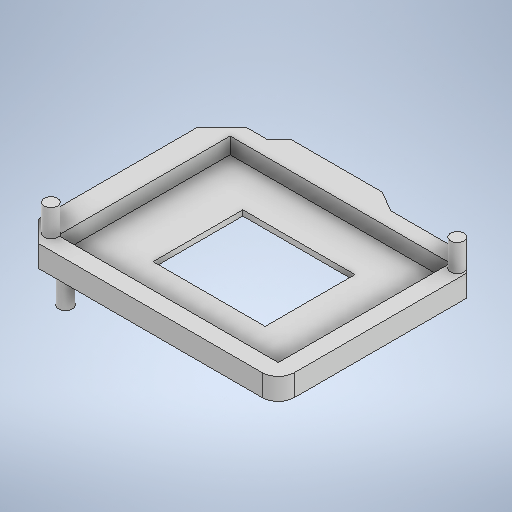
# Autodesk Inventor part: podstawka
Saved by Autodesk Inventor 2025.1 (Build 291241000, 241)
## iProperties
Created: 2024-10-24
Part Number: podstawka
Material: Ogólny
Document SubType Name: Modeling
Designer: PC
Density: 1 g/cm^3
Appearance: Domyślna
Author: PC
Autodesk Inventor part; units mm, degrees
ref_plane "YZ Plane" through (0, 0, 0) normal (1, 0, 0) x (0, 1, 0)
ref_plane "XZ Plane" through (0, 0, 0) normal (0, 1, 0) x (-1, 0, 0)
ref_plane "XY Plane" through (0, 0, 0) normal (0, 0, 1) x (1, 0, 0)
sketch "Szkic1" plane through (0, 0, 0) normal (0, 1, 0) x (-1, 0, 0)
  line L0 (-3.1297, -7.0475) -> (-3.1297, 9.5525)
  line L1 (17.6103, -7.0475) -> (-3.1297, -7.0475)
  line L2 (17.6103, 9.5525) -> (17.6103, -7.0475)
  line L3 (-3.1297, 9.5525) -> (17.6103, 9.5525)
  circle A0 centre (24.5703, 18.7775) radius 1.3
  circle A1 centre (-10.1297, -16.4225) radius 0.8
  line L4 (21.3203, -19.7725) -> (4.5808, -19.7725)
  line L5 (-16.2297, -14.5725) -> (-16.2297, 17.2275)
  line L6 (-13.2297, 20.2275) -> (28.0203, 20.2275)
  line L7 (32.0203, 16.2275) -> (32.0203, -13.0725)
  circle A2 centre (24.5703, 18.7775) radius 1.25
  line L8 (32.0203, 16.2275) -> (28.0203, 20.2275)
  arc A3 (-13.2297, 20.2275) -> (-16.2297, 17.2275) centre (-13.2297, 17.2275) ccw
  line L9 (4.5808, -19.7725) -> (0.7703, -17.5725)
  line L10 (0.7703, -17.5725) -> (-13.2297, -17.5725)
  line L11 (-13.2297, -17.5725) -> (-16.2297, -14.5725)
  line L12 (21.3203, -19.7725) -> (23.5203, -17.5725)
  line L13 (23.5203, -17.5725) -> (27.5203, -17.5725)
  line L14 (27.5203, -17.5725) -> (32.0203, -13.0725)
  line L15 (-13.1297, 17.1275) -> (27.6003, 17.1275)
  line L16 (27.6003, 17.1275) -> (27.6003, -14.6925)
  line L17 (27.6003, -14.6925) -> (-13.1297, -14.6925)
  line L18 (-13.1297, -14.6925) -> (-13.1297, 17.1275)
  circle A4 centre (28.5703, 17.4775) radius 1.25
  circle A5 centre (-14.5797, -14.5225) radius 1.25
  point P0 (0, 0)
  point P1 (-27.8297, -19.2225)
  point P2 (-15.1874, -15.6149)
  point P3 (-15.6721, -15.1301)
  point P4 (27.6003, 16.6891)
  point P5 (27.3703, 17.1275)
  dimension "d0" = 48.25
  dimension "d1" = 2.5
  dimension "d2" = 1.45
  dimension "d3" = 4
  dimension "d4" = 4
  dimension "d5" = 3
  dimension "d6" = 40
  dimension "d7" = 30
  dimension "d8" = 3
  dimension "d9" = 3
  dimension "d10" = 4.5
  dimension "d11" = 4.5
  dimension "d12" = 17
  dimension "d13" = 2.2
  dimension "d14" = 45
  dimension "d15" = 10.7
  dimension "d16" = 3.1
  dimension "d17" = 3.1
  dimension "d18" = 40.73
  dimension "d19" = 31.82
  dimension "d20" = 11.6
  dimension "d27" = 2.75
  dimension "d28" = 3.45
  dimension "d29" = 1.65
  dimension "d30" = 3.05
  dimension "d31" = 2.5
  dimension "d32" = 2.5
  constraints: 38 end point, 6 centre point, 5 horizontal, 4 parallel, 2 perpendicular, 2 point on circle, 2 point on line, 2 tangent, 2 vertical, 1 coincident, 9 other
  measures "d0" distance between parallel lines of L7 L5
  measures "d1" diameter of A2
  measures "d2" distance from line of L6 A2.centre
  measures "d3" distance from line of L6.end L7
  measures "d4" distance from line of L7.start L6
  measures "d5" radius of A3
  measures "d6" distance between parallel lines of L6 L4
  measures "d7" angle of L10 L9
  measures "d8" horizontal distance of L5.start L10.end
  measures "d9" horizontal distance of L5.start L10.end
  measures "d10" horizontal distance of L7.end L13.end
  measures "d11" horizontal distance of L7.end L13.end
  measures "d12" horizontal distance of L5.start L9.end
  measures "d13" distance between parallel lines of L10 L4
  measures "d14" angle of L13 L12
  measures "d15" distance from line of L7 L4.start
  measures "d16" distance between parallel lines of L15 L6
  measures "d17" distance between parallel lines of L5 L18
  measures "d18" distance of L15.start L15.end
  measures "d19" distance of L17.end L15.start
  measures "d20" distance from line of point (-27.83, -19.223) L5
  measures "d27" distance from line of L6 A4.centre
  measures "d28" distance from line of L7 A4.centre
  measures "d29" distance from line of L5 A5.centre
  measures "d30" distance from line of L10 A5.centre
  measures "d31" diameter of A4
  measures "d32" diameter of A5
extrude "Wyciągnięcie proste1" add sketch "Szkic1" along normal blind 4 contours A0 | A1 | L4 L9 L10 L11 A5 L5 A3 L6 L8 L7 L14 L13 L12 | L11 A5 | A2 | A4 L16 L15 picked at (-14.8001, -14.1216) picked at (29.019, 17.6576)
extrude "Wyciągnięcie proste2" add sketch "Szkic1" along normal blind 1 contours L15 A4 L16 L17 L18 | L15 L16 A4 picked at (27.5683, 16.8804)
extrude "Wyciągnięcie proste3" add sketch "Szkic1" against normal blind 4.8 contours A0 | A1 | A2
extrude "Wyciągnięcie proste4" add sketch "Szkic1" along normal blind 9 contours L11 A5 | A4 L16 L15 | L15 L16 A4 picked at (-14.8001, -14.1216)
